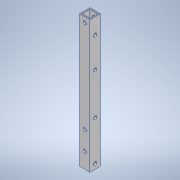
# Autodesk Inventor part: 上下直動9x9_2
Saved by Autodesk Inventor 2020.3 (Build 243373000, 373)
## iProperties
Created: 2020-07-05
Part Number: 上下直動9x9_2
Material: アルミニウム 6061
Document SubType Name: Modeling
Designer: totot
Density: 2.7 g/cm^3
Appearance: アルミニウム - フラット
Mass: 9.83397 g
Surface Area: 62.8095 cm^2
Volume: 3.64221 cm^3
Author: totot
Autodesk Inventor part; units mm, degrees
ref_plane "YZ Plane" through (0, 0, 0) normal (1, 0, 0) x (0, 1, 0)
ref_plane "XZ Plane" through (0, 0, 0) normal (0, 1, 0) x (-1, 0, 0)
ref_plane "XY Plane" through (0, 0, 0) normal (0, 0, 1) x (1, 0, 0)
sketch "スケッチ1" plane through (0, 0, 0) normal (0, 1, 0) x (-1, 0, 0)
  line L0 (0, 0) -> (-9, 0)
  line L1 (-9, 0) -> (-9, -9)
  line L2 (-9, -9) -> (0, -9)
  line L3 (0, -9) -> (0, 0)
  line L4 (-1.2, -1.2) -> (-7.8, -1.2)
  line L5 (-7.8, -1.2) -> (-7.8, -7.8)
  line L6 (-7.8, -7.8) -> (-1.2, -7.8)
  line L7 (-1.2, -7.8) -> (-1.2, -1.2)
  dimension "d0" = 9
  dimension "d1" = 9
  dimension "d2" = 6.6
  dimension "d3" = 6.6
  dimension "d4" = 1.2
  dimension "d5" = 1.2
  constraints: 16 end point, 4 parallel, 2 horizontal, 2 perpendicular
  measures "d0" distance of L2.end L1.end
  measures "d1" distance of L1.end L0.end
  measures "d2" distance of L6.end L5.end
  measures "d3" distance of L5.end L4.end
  measures "d4" distance between parallel lines of L0 L4
  measures "d5" distance between parallel lines of L7 L3
extrude "押し出し1" add sketch "スケッチ1" along normal blind 113.5
sketch "スケッチ2" plane through (0, 0, 0) normal (0, 0, 1) x (1, 0, 0)
  line L0 (0, 0) -> (9, 0) projected
  line L1 (0, 0) -> (0, 113.5) projected
  point P0 (4.5, 29.5)
  point P1 (4.5, 13.5)
  dimension "d8" = 13.5
  dimension "d9" = 4.5
  dimension "d10" = 16
  dimension "d11" = 4.5
  measures "d8" distance from line of L0 point (4.5, 13.5)
  measures "d9" distance from line of L1 point (4.5, 13.5)
  measures "d10" distance of point (4.5, 13.5) point (4.5, 29.5)
  measures "d11" distance from line of L1 point (4.5, 29.5)
hole "穴1" at (4.5, 29.5, 0) at (4.5, 13.5, 0) direction (0, 0, -1) diameter 3 end through all
sketch "スケッチ3" plane through (0, 0, -9) normal (-1, 0, 0) x (0, 0, 1)
  line L0 (0, 0) -> (9, 0) projected
  line L1 (0, 0) -> (0, 113.5) projected
  point P0 (4.5, 4.5)
  point P1 (4.5, 74)
  dimension "d19" = 4.5
  dimension "d20" = 4.5
  dimension "d21" = 4.5
  dimension "d22" = 69.5
  measures "d19" distance from line of L0 point (4.5, 4.5)
  measures "d20" distance from line of point (4.5, 4.5) L1
  measures "d21" distance from line of point (4.5, 74) L1
  measures "d22" distance of point (4.5, 74) point (4.5, 4.5)
hole "穴2" at (0, 4.5, -4.5) at (0, 74, -4.5) direction (1, 0, 0) diameter 3 end through all
sketch "スケッチ4" plane through (0, 0, -9) normal (-1, 0, 0) x (0, 0, 1)
  line L0 (0, 113.5) -> (9, 113.5) projected
  line L1 (0, 0) -> (0, 113.5) projected
  point P0 (9, 0)
  point P1 (4.5, 100)
  dimension "d30" = 13.5
  dimension "d31" = 4.5
  measures "d30" distance from line of point (4.5, 100) L0
  measures "d31" distance from line of point (4.5, 100) L1
hole "穴3" at (0, 100, -4.5) direction (1, 0, 0) diameter 3 end through all
sketch "スケッチ5" plane through (9, 0, -9) normal (0, 0, -1) x (-1, 0, 0)
  line L0 (0, 113.5) -> (9, 113.5) projected
  line L1 (9, 0) -> (9, 113.5) projected
  point P0 (4.5, 109)
  dimension "d39" = 4.5
  dimension "d40" = 4.5
  measures "d39" distance from line of L0 point (4.5, 109)
  measures "d40" distance from line of L1 point (4.5, 109)
hole "穴4" at (4.5, 109, -9) direction (0, 0, 1) diameter 3 end through all
sketch "スケッチ6" plane through (9, 0, 0) normal (1, 0, 0) x (0, 0, -1)
  line L0 (0, 0) -> (0, 113.5) projected
  circle A0 centre (4.5, 4.5) radius 1.5 projected
  point P0 (4.5, 38.5)
  dimension "d48" = 4.5
  dimension "d49" = 34
  measures "d48" distance from line of L0 point (4.5, 38.5)
  measures "d49" distance of point (4.5, 38.5) A0.centre
hole "穴5" at (9, 38.5, -4.5) direction (-1, 0, 0) diameter 3 end through all
equation "\"d11\" = d9"
equation "\"d21\" = d19"
equation "\"d39\" = d40"
